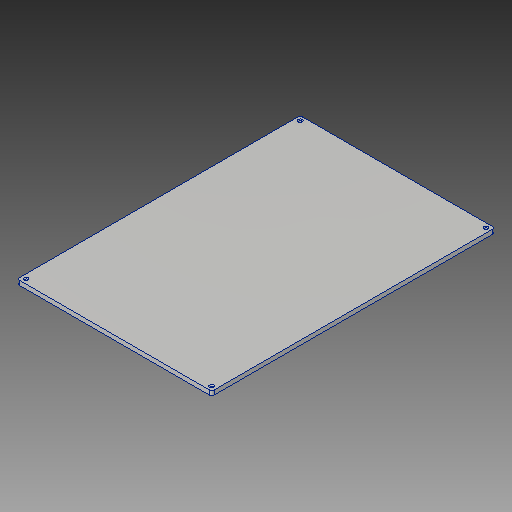
# Autodesk Inventor part: Bed Plate
Saved by Autodesk Inventor 2019 (Build 230136000, 136)
## iProperties
Created: 2018-10-07
Part Number: Bed Plate
Material: Aluminum 6061
Document SubType Name: Sheet Metal
Designer: Ax
Density: 2.7 g/cm^3
Sheet Metal Rule: Default_mm
Appearance: Aluminum - Flat
Flat Pattern Width: 22 cm
Flat Pattern Length: 32 cm
Flat Pattern Area: 704 cm^2
Sheet Metal Width: 220.000 mm
Sheet Metal Length: 320.000 mm
Sheet Metal Area: 70400.000 mm^2
Mass: 949.852 g
Surface Area: 1462.74 cm^2
Volume: 351.797 cm^3
Project: AX-01 CoreXY
Author: Ax
Autodesk Inventor part; units mm, degrees
ref_plane "YZ Plane" through (0, 0, 0) normal (1, 0, 0) x (0, 1, 0)
ref_plane "XZ Plane" through (0, 0, 0) normal (0, 1, 0) x (-1, 0, 0)
ref_plane "XY Plane" through (0, 0, 0) normal (0, 0, 1) x (1, 0, 0)
sketch "Sketch1" plane through (0, 0, 0) normal (0, 1, 0) x (-1, 0, 0)
  line L0 (-110, 160) -> (110, 160)
  line L1 (110, 160) -> (110, -160)
  line L2 (110, -160) -> (-110, -160)
  line L3 (-110, -160) -> (-110, 160)
  line L4 (-110, 160) -> (110, -160) construction
  line L5 (110, 160) -> (-110, -160) construction
  point P0 (0, 0)
  dimension "d0" = 220
  dimension "d1" = 320
  measures "d0" distance of L1.end L2.end
  measures "d1" distance of L0.end L1.end
extrude "Plate1" add sketch "Sketch1" along normal blind 5
fillet "Fillet1" radius 3 4 edges at (110, 2.5, 160) (-110, 2.5, 160) (110, 2.5, -160) (-110, 2.5, -160)
sketch "Sketch2" plane through (0, 5, 0) normal (0, 1, 0) x (1, 0, 0)
  line L0 (105, 155) -> (-105, 155) construction
  line L1 (-105, 155) -> (-105, -155) construction
  line L2 (-105, -155) -> (105, -155) construction
  line L3 (105, -155) -> (105, 155) construction
  line L4 (105, 155) -> (-105, -155) construction
  line L5 (-105, 155) -> (105, -155) construction
  circle A0 centre (105, -155) radius 1.6
  circle A1 centre (-105, -155) radius 1.6
  circle A2 centre (-105, 155) radius 1.6
  circle A3 centre (105, 155) radius 1.6
  point P0 (0, 0)
  dimension "d4" = 310
  dimension "d5" = 210
  dimension "d6" = 3.2
  constraints: 12 end point, 4 centre point, 4 coincident, 3 equal radius, 2 midpoint, 2 parallel, 1 horizontal, 1 perpendicular
  measures "d4" distance of L0.end L1.end
  measures "d5" distance of L1.end L2.end
  measures "d6" diameter of A0
hole "Hole1" at (105, 5, 155) at (-105, 5, 155) at (-105, 5, -155) at (105, 5, -155) direction (0, -1, 0) diameter 3 depth 8.8 countersink diameter 5 countersink angle 90
equation "\"d16\" = Thickness"
equation "\"TransitionRadius\" = BendRadius"
equation "\"JacobiRadiusSize\" = BendRadius"
equation "\"d2\" = BendRadius"
equation "\"Thickness\" = 5"
equation "\"BendRadius\" = 0.8"
body "Solid1"
